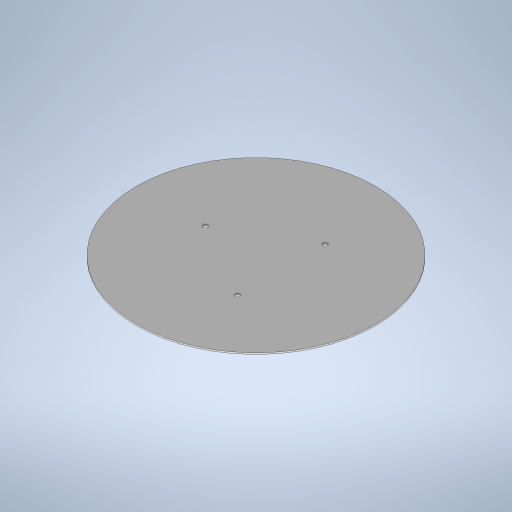
# Autodesk Inventor part: basespacer2
Saved by Autodesk Inventor 2024 (Build 280153000, 153)
## iProperties
Created: 2025-08-23
Part Number: basespacer2
Material: 一般
Document SubType Name: Modeling
Designer: tanoue_kota
Density: 1 g/cm^3
Appearance: 既定
Author: tanoue_kota
Autodesk Inventor part; units mm, degrees
ref_plane "YZ Plane" through (0, 0, 0) normal (1, 0, 0) x (0, 1, 0)
ref_plane "XZ Plane" through (0, 0, 0) normal (0, 1, 0) x (-1, 0, 0)
ref_plane "XY Plane" through (0, 0, 0) normal (0, 0, 1) x (1, 0, 0)
sketch "スケッチ1" plane through (0, 0, 0) normal (0, 1, 0) x (-1, 0, 0)
  circle A0 centre (0, 0) radius 86.2565
  dimension "d0" = 172.513
  constraints: 1 centre point, 1 coincident
  measures "d0" diameter of A0
extrude "押し出し1" add sketch "スケッチ1" along normal blind 1
sketch "スケッチ2" plane through (0, 1, 0) normal (0, 1, 0) x (1, 0, 0)
  circle A0 centre (0, 0) radius 36.5
  point P0 (-36.5, 0)
  point P1 (18.25, -31.6099)
  point P2 (18.25, 31.6099)
  dimension "d3" = 73
  dimension "d6" = 360
  constraints: 1 coincident, 1 horizontal alignment, 6 other
hole "穴1" at (-36.5, 1, 0) at (18.25, 1, 31.6099) at (18.25, 1, -31.6099) direction (0, -1, 0) diameter 3.3 end through all
